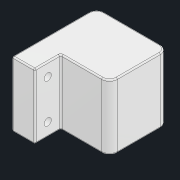
# Autodesk Inventor part: scara-base24
Saved by Autodesk Inventor 2022 (Build 260153000, 153)
## iProperties
Created: 2021-10-30
Part Number: scara-base24
Material: ABS プラスチック
Document SubType Name: Modeling
Designer: Yuta Kage
Density: 1.06 g/cm^3
Appearance: 滑らか - 白
Author: Yuta Kage
Autodesk Inventor part; units mm, degrees
ref_plane "YZ Plane" through (0, 0, 0) normal (1, 0, 0) x (0, 1, 0)
ref_plane "XZ Plane" through (0, 0, 0) normal (0, 1, 0) x (-1, 0, 0)
ref_plane "XY Plane" through (0, 0, 0) normal (0, 0, 1) x (1, 0, 0)
sketch "スケッチ1" plane through (0, 0, 0) normal (0, 1, 0) x (-1, 0, 0)
  line L0 (22.5, 17.5) -> (-22.5, 17.5) construction
  line L1 (-22.5, 17.5) -> (-22.5, -17.5) construction
  line L2 (-22.5, -17.5) -> (22.5, -17.5) construction
  line L3 (22.5, -17.5) -> (22.5, 17.5) construction
  line L4 (22.5, 17.5) -> (-22.5, -17.5) construction
  line L5 (-22.5, 17.5) -> (22.5, -17.5) construction
  line L6 (27.5, 22.5) -> (-27.5, 22.5)
  line L7 (-27.5, 22.5) -> (-27.5, -22.5)
  line L8 (-27.5, -22.5) -> (27.5, -22.5)
  line L9 (27.5, -22.5) -> (27.5, 22.5)
  line L10 (10, 42.5) -> (27.5, 42.5)
  line L11 (27.5, 42.5) -> (27.5, 22.5)
  line L12 (27.5, 22.5) -> (10, 22.5)
  line L13 (10, 22.5) -> (10, 42.5)
  line L14 (10, 42.5) -> (27.5, 22.5) construction
  line L15 (27.5, 42.5) -> (10, 22.5) construction
  point P0 (0, 0)
  point P1 (0, 0)
  point P2 (18.75, 32.5)
  point P3 (10, 22.5)
  dimension "d0" = 45
  dimension "d1" = 35
  dimension "d2" = 5
  dimension "d4" = 20
  dimension "d5" = 10
  constraints: 32 end point, 6 parallel, 5 midpoint, 3 perpendicular, 2 horizontal, 3 other
  measures "d0" distance of L1.end L2.end
  measures "d1" distance of L2.end L0.start
  measures "d2" distance between parallel lines of L9 L3
  measures "d4" distance of L10.end L6.start
  measures "d5" distance from line of point (0, 0) L13
extrude "押し出し1" add sketch "スケッチ1" along normal blind 50
sketch "スケッチ2" plane through (-27.5, 0, -22.5) normal (-1, 0, 0) x (0, 0, 1)
  line L0 (0, 50) -> (65, 50) projected
  line L1 (65, 0) -> (65, 50) projected
  line L2 (0, 0) -> (65, 0) projected
  point P0 (22.5, 0)
  point P1 (55, 40)
  point P2 (55, 10)
  dimension "d8" = 10
  dimension "d9" = 10
  dimension "d24" = 10
  constraints: 1 vertical alignment
  measures "d8" distance from line of L0 point (55, 40)
  measures "d9" distance from line of L1 point (55, 40)
  measures "d24" distance from line of L2 point (55, 10)
hole "穴1" at (-27.5, 10, 32.5) at (-27.5, 40, 32.5) direction (1, 0, 0) diameter 5.5 end through all clearance for "Flat Head Machine Screw" size "M5" standard "Ansi Metric M Profile"
sketch "スケッチ3" plane through (0, 0, 0) normal (0, -1, 0) x (1, 0, 0)
  line L0 (-23.5, 18.5) -> (23.5, 18.5)
  line L1 (23.5, 18.5) -> (23.5, -18.5)
  line L2 (23.5, -18.5) -> (-23.5, -18.5)
  line L3 (-23.5, -18.5) -> (-23.5, 18.5)
  line L4 (-23.5, 18.5) -> (23.5, -18.5) construction
  line L5 (23.5, 18.5) -> (-23.5, -18.5) construction
  point P0 (0, 0)
  dimension "d17" = 37
  dimension "d18" = 47
  constraints: 12 end point, 2 midpoint, 2 parallel, 1 horizontal, 1 perpendicular
  measures "d17" distance of L0.end L1.end
  measures "d18" distance of L1.end L2.end
extrude "押し出し2" cut sketch "スケッチ3" against normal blind 46
fillet "フィレット1" radius 2 8 edges at (23.5, 23, 18.5) (0, 46, 18.5) (23.5, 46, 0) (0, 46, -18.5) (-23.5, 46, 0) (-23.5, 23, 18.5) (-23.5, 23, -18.5) (23.5, 23, -18.5)
fillet "フィレット2" radius 6 3 edges at (27.5, 25, 22.5) (27.5, 25, -22.5) (-27.5, 25, -22.5)
fillet "フィレット4" radius 1 1 edges at (-10, 25, 22.5)
fillet "フィレット5" radius 1 22 edges at (-18.75, 0, 42.5) (-27.5, 25, 42.5) (-25.7426, 0, -20.7426) (0, 0, -22.5) (25.7426, 0, -20.7426) (27.5, 0, 0) (25.7426, 0, 20.7426) (6.25, 0, 22.5) (-9.7071, 0, 22.7929) (-10, 0, 33) (-27.5, 0, 13) (-10, 25, 42.5) (-18.75, 50, 42.5) (-25.7426, 50, -20.7426) (0, 50, -22.5) (25.7426, 50, -20.7426) (27.5, 50, 0) (25.7426, 50, 20.7426) (6.25, 50, 22.5) (-9.7071, 50, 22.7929) (-10, 50, 33) (-27.5, 50, 13)
chamfer "面取り1" distance 10 angle 10 8 edges at (23.5, 0, 0) (22.9142, 0, -17.9142) (0, 0, -18.5) (-22.9142, 0, -17.9142) (-23.5, 0, 0) (-22.9142, 0, 17.9142) (0, 0, 18.5) (22.9142, 0, 17.9142) measured on face at (-22.9142, 0.5, -17.9142) measured on face at (22.9142, 0.5, 17.9142) measured on face at (0, 0.5, 18.5) measured on face at (22.9142, 0.5, -17.9142) measured on face at (0, 0.5, -18.5) measured on face at (-22.9142, 0.5, 17.9142) measured on face at (23.5, 0.5, 0) measured on face at (-23.5, 0.5, 0)
